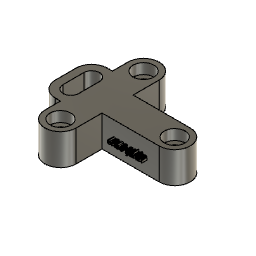
Model 16 (Autodesk Fusion 360 design; units mm, degrees)
Autodesk Fusion 360 part; units mm, degrees
sketch "Sketch1" plane through (0, 0, 0) normal (0, 0, 1) x (1, 0, 0)
  line L0 (0, 0) -> (70, 0) construction
  circle A0 centre (70, 0) radius 5
  circle A1 centre (70, 0) radius 10
  line L1 (0, 0) -> (0, 40) construction
  line L2 (0, 0) -> (0, -40) construction
  circle A2 centre (70, 0) radius 10
  circle A3 centre (70, 0) radius 5
  circle A4 centre (0, -40) radius 10
  circle A5 centre (0, -40) radius 5
  circle A6 centre (0, 40) radius 5
  circle A7 centre (0, 40) radius 10
  line L3 (0, 0) -> (-20, 0) construction
  line L4 (-20, 0) -> (-20, 10) construction
  line L5 (-20, 0) -> (-20, -10) construction
  line L6 (-35, 10) -> (-35, -10)
  line L7 (-12.5, 10) -> (-12.5, -10)
  line L8 (-27.5, 10) -> (-27.5, -10)
  line L9 (-20, -25) -> (-15, -25)
  line L10 (70, -15) -> (15, -15)
  line L11 (-15, 40) -> (-15, 25)
  line L12 (15, 40) -> (15, 25)
  line L13 (15, 25) -> (15, 15)
  line L14 (15, -40) -> (15, -15)
  line L15 (-15, -40) -> (-15, -25)
  line L16 (70, 15) -> (15, 15)
  arc A8 (-15, -40) -> (15, -40) centre (0, -40) ccw
  arc A9 (-12.5, 10) -> (-27.5, 10) centre (-20, 10) ccw
  arc A10 (-27.5, -10) -> (-12.5, -10) centre (-20, -10) ccw
  arc A11 (-20, 25) -> (-35, 10) centre (-20, 10) ccw
  arc A12 (-35, -10) -> (-20, -25) centre (-20, -10) ccw
  line L17 (-20, 25) -> (-15, 25)
  arc A13 (15, 40) -> (-15, 40) centre (0, 40) ccw
  arc A14 (70, -15) -> (70, 15) centre (70, 0) ccw
  arc A15 (70, -15) -> (70, 15) centre (70, 0) ccw
  point P0 (0, 40)
  dimension "d1" = 70
  dimension "d2" = 10
  dimension "d3" = 20
  dimension "d4" = 30
  dimension "d8" = 40
  dimension "d9" = 40
  dimension "d10" = 10
  dimension "d11" = 20
  dimension "d12" = 30
  dimension "d13" = 10
  dimension "d14" = 20
  dimension "d15" = 30
  dimension "d16" = 10
  dimension "d17" = 20
  dimension "d18" = 30
  dimension "d19" = 20
  dimension "d20" = 10
  dimension "d21" = 10
  dimension "d22" = 15
  dimension "d23" = 15
  constraint coincident L0.start L1.start
  constraint horizontal L0
  constraint coincident L0.end A0.centre
  constraint concentric A0 A1
  constraint concentric A1 A15
  constraint perpendicular L0 L1
  constraint perpendicular L0 L2
  constraint concentric A2 A3
  constraint concentric A2 A14
  constraint concentric A4 A5
  constraint concentric A6 A7
  constraint perpendicular L2 L3
  constraint perpendicular L3 L4
  constraint perpendicular L3 L5
  constraint coincident L4.end A9.centre
  constraint coincident L5.end A10.centre
  constraint tangent L7 A10
  constraint tangent L8 A10
  constraint tangent L16 A15
  constraint tangent L10 A14
  constraint perpendicular L2 L10
  constraint tangent L11 A13
  constraint perpendicular L11 L17
  constraint tangent L12 A13
  constraint perpendicular L13 L16
  constraint tangent L14 A8
  constraint perpendicular L10 L14
  constraint tangent L15 A8
  measures "d1" distance of L0.start L0.end
  measures "d2" diameter of A0
  measures "d3" diameter of A1
  measures "d4" diameter of A15
  measures "d8" distance of L0.start P0
  measures "d9" distance of L0.start L2.end
  measures "d10" diameter of A3
  measures "d11" diameter of A2
  measures "d12" diameter of A14
  measures "d13" diameter of A5
  measures "d14" diameter of A4
  measures "d15" diameter of A8
  measures "d16" diameter of A6
  measures "d17" diameter of A7
  measures "d18" diameter of A13
  measures "d19" distance of L0.start L3.end
  measures "d20" distance of L3.end L4.end
  measures "d21" distance of L3.end L5.end
  measures "d22" diameter of A9
  measures "d23" diameter of A10
extrude "Extrude1" add sketch "Sketch1" along normal blind 30 contours L6 L9 L10 L11 L12 L13 L14 L15 L16 A8 A11 A12 L17 A13 A14 A15
extrude "Extrude2" add sketch "Sketch1" along normal blind 20 contours A1 A2 | A4 | A7
ref_plane "WorkPlane1" through (42.5, -15, 15) normal (0, -1, 0) x (1, 0, 0)
sketch "Sketch2" plane through (42.5, -15, 15) normal (0, -1, 0) x (1, 0, 0)
  line L0 (-17.3651, -2.2192) -> (17.3567, -2.2836) construction
  line L1 (17.3567, -2.2836) -> (17.3651, 2.2192) construction
  line L2 (17.3651, 2.2192) -> (-17.3567, 2.2836) construction
  line L3 (-17.3567, 2.2836) -> (-17.3651, -2.2192) construction
  text T0 "enes şahin" font "Arial" height 5 align left top in box 34.7219 x 4.5028 at (-17.3651, -2.2192) x (0.999998, -0.001856) y (0.001856, 0.999998) spacing 1
  constraint coincident origin
extrude "Extrude3" add sketch "Sketch2" along normal blind 5 text T0
